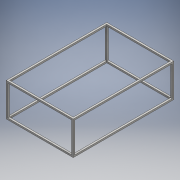
# Autodesk Inventor part: CubeSat Frame
Saved by Autodesk Inventor 2016 (Build 200138000, 138)
## iProperties
Created: 2015-12-21
Part Number: CubeSat Frame
Material: Generic
Document SubType Name: Modeling
Designer: jonathan
Density: 1 g/cm^3
Appearance: Default
Author: jonathan
Autodesk Inventor part; units mm, degrees
ref_plane "YZ Plane" through (0, 0, 0) normal (1, 0, 0) x (0, 1, 0)
ref_plane "XZ Plane" through (0, 0, 0) normal (0, 1, 0) x (-1, 0, 0)
ref_plane "XY Plane" through (0, 0, 0) normal (0, 0, 1) x (1, 0, 0)
sketch "Sketch1" plane through (0, 0, 0) normal (0, 1, 0) x (-1, 0, 0)
  line L0 (0, 0) -> (200, 0)
  line L1 (200, 0) -> (200, -100)
  line L2 (200, -100) -> (0, -100)
  line L3 (0, -100) -> (0, 0)
  point P0 (100, -50)
  dimension "d0" = 100
  dimension "d1" = 200
  constraints: 8 end point, 2 parallel, 1 horizontal, 1 perpendicular
  measures "d0" distance of L0.end L1.end
  measures "d1" distance of L1.end L2.end
extrude "Extrusion1" add sketch "Sketch1" along normal blind 300
sketch "Sketch3" plane through (0, 0, 0) normal (0, 0, 1) x (1, 0, 0)
  line L0 (-200, 300) -> (0, 300) projected
  line L1 (-200, 300) -> (0, 300)
  line L2 (0, 300) -> (0, 0)
  line L3 (0, 0) -> (-200, 0)
  line L4 (-200, 0) -> (-200, 300)
  line L5 (-195, 295) -> (-5, 295)
  line L6 (-5, 295) -> (-5, 5)
  line L7 (-5, 5) -> (-195, 5)
  line L8 (-195, 5) -> (-195, 295)
  line L9 (-195, 295) -> (-5, 5) construction
  line L10 (-5, 295) -> (-195, 5) construction
  point P0 (-100, 150)
  dimension "d8" = 5
  dimension "d9" = 5
  dimension "d10" = 5
  dimension "d11" = 5
  constraints: 20 end point, 4 parallel, 2 horizontal, 2 midpoint, 2 perpendicular
  measures "d8" distance between parallel lines of L8 L4
  measures "d9" distance between parallel lines of L3 L7
  measures "d10" distance between parallel lines of L2 L6
  measures "d11" distance between parallel lines of L0 L5
extrude "Extrusion2" cut sketch "Sketch3" against normal through all contours L5 L6 L7 L8
sketch "Sketch4" plane through (0, 0, 0) normal (1, 0, 0) x (0, 1, 0)
  line L0 (0, 0) -> (300, 0) projected
  line L1 (0, -100) -> (300, -100) projected
  line L2 (0, 0) -> (300, 0)
  line L3 (300, 0) -> (300, -100)
  line L4 (300, -100) -> (0, -100)
  line L5 (0, -100) -> (0, 0)
  line L6 (295, -5) -> (5, -5)
  line L7 (5, -5) -> (5, -95)
  line L8 (5, -95) -> (295, -95)
  line L9 (295, -95) -> (295, -5)
  line L10 (295, -5) -> (5, -95) construction
  line L11 (5, -5) -> (295, -95) construction
  point P0 (150, -50)
  dimension "d14" = 5
  dimension "d15" = 5
  dimension "d16" = 5
  dimension "d17" = 5
  constraints: 20 end point, 4 parallel, 2 horizontal, 2 midpoint, 2 perpendicular
  measures "d14" distance between parallel lines of L0 L6
  measures "d15" distance between parallel lines of L5 L7
  measures "d16" distance between parallel lines of L1 L8
  measures "d17" distance between parallel lines of L3 L9
extrude "Extrusion3" cut sketch "Sketch4" against normal through all contours L9 L8 L7 L6
sketch "Sketch6" plane through (0, 0, 0) normal (0, 1, 0) x (-1, 0, 0)
  line L0 (195, -5) -> (5, -5)
  line L1 (5, -5) -> (5, -95)
  line L2 (5, -95) -> (195, -95)
  line L3 (195, -95) -> (195, -5)
  line L4 (195, -5) -> (5, -95) construction
  line L5 (5, -5) -> (195, -95) construction
  line L6 (200, 0) -> (200, -100) projected
  line L7 (0, 0) -> (200, 0) projected
  line L8 (0, -100) -> (0, 0) projected
  line L9 (200, -100) -> (0, -100) projected
  point P0 (100, -50)
  dimension "d20" = 5
  dimension "d21" = 5
  dimension "d22" = 5
  dimension "d23" = 5
  constraints: 12 end point, 2 midpoint, 2 parallel, 1 horizontal, 1 perpendicular
  measures "d20" distance between parallel lines of L6 L3
  measures "d21" distance between parallel lines of L0 L7
  measures "d22" distance between parallel lines of L8 L1
  measures "d23" distance between parallel lines of L9 L2
extrude "Extrusion4" cut sketch "Sketch6" along normal through all contours L3 L2 L1 L0
body "Solid1"
